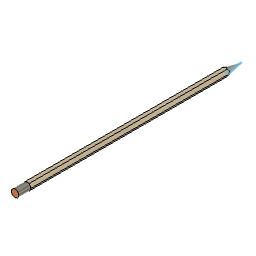
Pencil v3 (Autodesk Fusion 360 design; units mm, degrees)
Autodesk Fusion 360 part; units mm, degrees
sketch "Sketch1" plane through (0, 0, 0) normal (0, 1, 0) x (1, 0, 0)
  line L0 (1.775, -3.0744) -> (3.55, 0)
  line L1 (3.55, 0) -> (1.775, 3.0744)
  line L2 (1.775, 3.0744) -> (-1.775, 3.0744)
  line L3 (-1.775, 3.0744) -> (-3.55, 0)
  line L4 (-3.55, 0) -> (-1.775, -3.0744)
  line L5 (-1.775, -3.0744) -> (1.775, -3.0744)
  circle A0 centre (0, 0) radius 3.55
  dimension "d6" = 3.55
  dimension "d8" = 7.1
  constraint coincident A0.centre origin
  constraint horizontal L2
  measures "d6" distance of L0.start A0.centre
  measures "d8" diameter of A0
extrude "Extrude1" add sketch "Sketch1" along normal blind 190
sketch "Sketch2" plane through (0, 0, 0) normal (0, 0, 1) x (1, 0, 0)
  line L0 (0, 190) -> (0, 205.8333)
  line L1 (0, 205.8333) -> (3.5149, 190)
  line L2 (0, 190) -> (3.5149, 190)
  dimension "d11" = 15.8333
  constraint vertical L0
  constraint perpendicular L0 L2
  measures "d11" distance of L0.start L0.end
revolve "Revolve1" add sketch "Sketch2" angle 360 about axis through (0, 190, 0) along (0, 1, 0)
extrude "Extrude2" cut sketch "Sketch1" along normal blind 205 contours L5 A0 | L0 A0 | L1 A0 | L4 A0 | L2 A0 | L3 A0
sketch "Sketch3" plane through (0, 0, 0) normal (1, 0, 0) x (0, 1, 0)
extrude "Extrude3" add sketch "Sketch1" against normal blind 11.7
equation "width = 7.1 mm"
equation "tip_diameter = 2.4 mm"
equation "eraser_holder_height = 11.7 mm"
equation "eraser_height = 4.7 mm"
equation "height = 190 mm"
equation "d6 = width / 2"
equation "d8 = width"
equation "d9 = height"
equation "d11 = height / 12"
equation "d15 = eraser_holder_height * -1"
